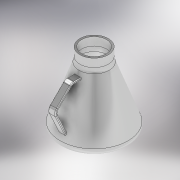
# Autodesk Inventor part: 特征3
Saved by Autodesk Inventor 2020 (Build 240168000, 168)
## iProperties
Created: 2021-03-24
Part Number: 特征3
Material: 镍铜合金 400
Document SubType Name: Modeling
Designer: Luorily
Density: 8.83 g/cm^3
Appearance: 铬 - 抛光
Author: Luorily
Autodesk Inventor part; units mm, degrees
ref_plane "YZ Plane" through (0, 0, 0) normal (1, 0, 0) x (0, 1, 0)
ref_plane "XZ Plane" through (0, 0, 0) normal (0, 1, 0) x (-1, 0, 0)
sketch "草图1" plane through (0, 0, 0) normal (0, 0, 1) x (1, 0, 0)
  line L0 (0, 0) -> (60, 0)
  line L1 (60, 0) -> (60, -45)
  line L2 (60, -45) -> (127.93709, -45) construction
  line L3 (60, -45) -> (152.81241, -300)
  line L4 (152.81241, -300) -> (0, -300)
  line L5 (0, -300) -> (0, 0)
  dimension "d0" = 60
  dimension "d1" = 45
  dimension "d3" = 255
  dimension "d4" = 160
  constraints: 12 end point, 3 horizontal, 2 perpendicular
  measures "d0" distance of L0.start L0.end
  measures "d1" distance of L0.end L1.end
  measures "d3" vertical distance of L1.end L3.end
  measures "d4" angle of L3 L1
revolve "旋转1" add sketch "草图1" angle 360 about axis through (0, -300, 0) along (0, 1, 0)
fillet "圆角1" radius 20 1 edges at (-152.8124, -300, 0)
fillet "圆角2" radius 60 1 edges at (-60, -45, 0)
shell "抽壳1" thickness 8 removed faces 1 at (20.344473, 0, 12.200044)
sketch "草图2" plane through (0, 0, 0) normal (1, 0, 0) x (0, 1, 0)
  line L0 (-54.94159, 63.618443) -> (-273.159597, 143.043302)
  line L1 (-76.295083, 71.390479) -> (-76.295083, 99.106207)
  line L2 (-82.152947, 113.248343) -> (-137.103331, 168.198727)
  line L3 (-159.697832, 172.182747) -> (-244.53226, 132.623803)
  arc A0 (-76.295083, 106.147838) -> (-77.173763, 108.269158) centre (-79.295083, 106.147838) ccw
  arc A1 (-145.520397, 176.615792) -> (-148.909572, 177.213395) centre (-147.641717, 174.494472) ccw
  arc A2 (-76.295083, 99.106207) -> (-82.152947, 113.248343) centre (-96.295083, 99.106207) ccw
  arc A3 (-137.103331, 168.198727) -> (-159.697832, 172.182747) centre (-151.245467, 154.056591) ccw
  point P0 (0, 0)
  point P1 (-76.295083, 107.390479)
  point P2 (-147.005761, 178.101157)
  dimension "d9" = 36
  dimension "d10" = 100
  dimension "d11" = 135
  dimension "d12" = 110
  dimension "d13" = 3
  dimension "d14" = 20
  constraints: 10 point on line, 8 point on circle, 8 tangent, 6 end point, 4 centre point, 2 equal radius, 1 vertical
  measures "d9" distance of L1.start point (-76.295, 107.39)
  measures "d10" distance of point (-76.295, 107.39) point (-147.006, 178.101)
  measures "d11" angle of L2 L1
  measures "d12" angle of L3 L2
  measures "d13" radius of A0
  measures "d14" radius of A2
ref_plane "工作平面1" through (0, -137.103331, 168.198727) normal (0, -0.7071068, 0.7071068) x (1, 0, 0)
sketch "草图3" plane through (0, -137.103331, 168.198727) normal (0, -0.7071068, 0.7071068) x (1, 0, 0)
  line L0 (-12, 5) -> (12, 5)
  line L1 (15, 2) -> (15, -2)
  line L2 (12, -5) -> (-12, -5)
  line L3 (-15, -2) -> (-15, 2)
  arc A0 (-12, 5) -> (-15, 2) centre (-12, 2) ccw
  arc A1 (-15, -2) -> (-12, -5) centre (-12, -2) ccw
  arc A2 (12, -5) -> (15, -2) centre (12, -2) ccw
  arc A3 (15, 2) -> (12, 5) centre (12, 2) ccw
  point P0 (0, -21.987765)
  point P1 (0, 0)
  point P2 (0, 0)
  point P3 (0, 0)
  point P4 (15, 0)
  point P5 (0, 5)
  dimension "d15" = 3
  dimension "d16" = 30
  dimension "d17" = 10
  constraints: 8 end point, 8 point on circle, 8 tangent, 4 centre point, 3 equal radius, 2 midpoint, 2 parallel, 1 horizontal, 1 horizontal alignment, 1 perpendicular, 1 vertical alignment
  measures "d15" radius of A0
  measures "d16" distance between parallel lines of L1 L3
  measures "d17" distance between parallel lines of L0 L2
sweep "扫掠1" add profiles "草图3" path "草图2" path curves L3 A3 L2 A2 L1
sketch "草图5" plane through (12, -71.295083, 71.390479) normal (0, 0, -1) x (-1, 0, 0)
  spline S0 degree 2 poles (26.317143, -8.905479) (12, -1.170766) (-2.317143, -8.905479) knots 0 0 0 1 1 1 weights 1 1.01991131 1
  arc A0 (26.317143, -8.905479) -> (27, -7) centre (24, -7) ccw
  line L0 (27, -7) -> (27, -3)
  arc A1 (27, -3) -> (24, 0) centre (24, -3) ccw
  line L1 (24, 0) -> (0, 0)
  arc A2 (0, 0) -> (-3, -3) centre (0, -3) ccw
  line L2 (-3, -3) -> (-3, -7)
  arc A3 (-3, -7) -> (-2.317143, -8.905479) centre (0, -7) ccw
  point P0 (12, 71.295083)
  constraints: 1 horizontal alignment
extrude "拉伸2" add sketch "草图5" along normal up to surface
sketch "草图6" plane through (-12, -246.645352, 137.155342) normal (0, -0.9063078, -0.4226183) x (1, 0, 0)
  ellipse E0 centre (12, -130.101659) end of major axis (12, -5) minor radius 111.735678 (27, -6.132405) -> (-3, -6.132405) ccw
  line L0 (27, -6.132405) -> (27, -3)
  arc A0 (27, -3) -> (24, 0) centre (24, -3) ccw
  line L1 (24, 0) -> (0, 0)
  arc A1 (0, 0) -> (-3, -3) centre (0, -3) ccw
  line L2 (-3, -3) -> (-3, -6.132405)
  point P0 (12, -228.541785)
  constraints: 1 other
extrude "拉伸3" add sketch "草图6" along normal up to surface
